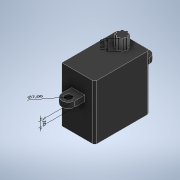
# Autodesk Inventor part: servo
Saved by Autodesk Inventor 2021 (Build 250183000, 183)
## iProperties
Created: 2021-02-24
Part Number: servo
Material: Rubber
Document SubType Name: Modeling
Designer: WASHINGTON
Density: 0.93 g/cm^3
Appearance: Rubber - Black
Author: WASHINGTON
Autodesk Inventor part; units mm, degrees
ref_plane "YZ Plane" through (0, 0, 0) normal (1, 0, 0) x (0, 1, 0)
ref_plane "XZ Plane" through (0, 0, 0) normal (0, 1, 0) x (-1, 0, 0)
ref_plane "XY Plane" through (0, 0, 0) normal (0, 0, 1) x (1, 0, 0)
sketch "Sketch1" plane through (0, 0, 0) normal (0, 1, 0) x (-1, 0, 0)
  line L0 (15, 25) -> (-15, 25)
  line L1 (-15, 25) -> (-15, -25)
  line L2 (-15, -25) -> (15, -25)
  line L3 (15, -25) -> (15, 25)
  circle A0 centre (0, -34) radius 3.5
  arc A1 (-6, -34) -> (6, -34) centre (0, -34) ccw
  line L4 (6, -34) -> (6, -25)
  line L5 (-6, -34) -> (-6, -25)
  line L6 (21.3749, 0) -> (-33.1106, 0) construction
  circle A2 centre (0, 34) radius 3.5
  arc A3 (6, 34) -> (-6, 34) centre (0, 34) ccw
  line L7 (6, 34) -> (6, 25)
  line L8 (-6, 34) -> (-6, 25)
  point P0 (0, 0)
  dimension "d0" = 25
  dimension "d1" = 25
  dimension "d2" = 15
  dimension "d3" = 15
  dimension "d4" = 7
  dimension "d5" = 12
  dimension "d6" = 9
  dimension "d7" = 34
  dimension "d8" = 12
  dimension "d9" = 34
  constraints: 18 end point, 6 symmetric about line, 4 centre point, 4 point on circle, 3 perpendicular, 2 coincident, 2 horizontal, 2 parallel, 2 point on line, 1 tangent, 2 other
  measures "d0" vertical distance of point (0, 0) L0.start
  measures "d1" distance from line of point (0, 0) L2
  measures "d2" horizontal distance of point (0, 0) L2.end
  measures "d3" horizontal distance of point (0, 0) L1.end
  measures "d4" diameter of A0
  measures "d5" diameter of A1
  measures "d6" distance from line of L2 A1.centre
  measures "d7" distance of point (0, 0) A0.centre
  measures "d8" distance between parallel lines of L5 L4
  measures "d9" distance of point (0, 0) A3.centre
extrude "Extrusion1" add sketch "Sketch1" along normal mid plane 5
sketch "Sketch2" plane through (0, 2.5, 0) normal (0, 1, 0) x (1, 0, 0)
  line L0 (-15, -25) -> (-15, 25) projected
  line L1 (6, 25) -> (15, 25) projected
  line L2 (-15, -25) -> (15, -25)
  line L3 (15, -25) -> (15, 25)
  line L4 (15, 25) -> (-15, 25)
  line L5 (-15, 25) -> (-15, -25)
  point P0 (0, 0)
  constraints: 8 end point, 2 parallel, 1 horizontal, 1 perpendicular
extrude "Extrusion2" add sketch "Sketch2" along normal blind 15 and the other way blind 35
sketch "Sketch3" plane through (0, 17.5, 0) normal (0, 1, 0) x (1, 0, 0)
  circle A0 centre (0, 15) radius 4
  line L0 (15, 25) -> (-15, 25) projected
  line L1 (-4, 15) -> (-5, 15) construction
  line L2 (-5, 15) -> (-5, 15.5)
  line L3 (-5, 15.5) -> (-3.8219, 16.1802)
  line L4 (-5, 15) -> (-5, 14.5)
  line L5 (-5, 14.5) -> (-3.8219, 13.8198)
  line L6 (-3.8891, 11.818) -> (-3.537, 13.132)
  line L7 (-3.5355, 11.4645) -> (-3.8891, 11.818)
  line L8 (-3.5355, 11.4645) -> (-3.182, 11.1109)
  line L9 (-3.182, 11.1109) -> (-1.868, 11.463)
  line L10 (-0.5, 10) -> (-1.1802, 11.1781)
  line L11 (0, 10) -> (-0.5, 10)
  line L12 (0, 10) -> (0.5, 10)
  line L13 (0.5, 10) -> (1.1802, 11.1781)
  line L14 (3.182, 11.1109) -> (1.868, 11.463)
  line L15 (3.5355, 11.4645) -> (3.182, 11.1109)
  line L16 (3.5355, 11.4645) -> (3.8891, 11.818)
  line L17 (3.8891, 11.818) -> (3.537, 13.132)
  line L18 (5, 14.5) -> (3.8219, 13.8198)
  line L19 (5, 15) -> (5, 14.5)
  line L20 (5, 15) -> (5, 15.5)
  line L21 (5, 15.5) -> (3.8219, 16.1802)
  line L22 (3.8891, 18.182) -> (3.537, 16.868)
  line L23 (3.5355, 18.5355) -> (3.8891, 18.182)
  line L24 (3.5355, 18.5355) -> (3.182, 18.8891)
  line L25 (3.182, 18.8891) -> (1.868, 18.537)
  line L26 (0.5, 20) -> (1.1802, 18.8219)
  line L27 (0, 20) -> (0.5, 20)
  line L28 (0, 20) -> (-0.5, 20)
  line L29 (-0.5, 20) -> (-1.1802, 18.8219)
  line L30 (-3.182, 18.8891) -> (-1.868, 18.537)
  line L31 (-3.5355, 18.5355) -> (-3.182, 18.8891)
  line L32 (-3.5355, 18.5355) -> (-3.8891, 18.182)
  line L33 (-3.8891, 18.182) -> (-3.537, 16.868)
  point P0 (0, 0)
  dimension "d16" = 8
  dimension "d17" = 10
  dimension "d18" = 15
  dimension "d19" = 120
  dimension "d20" = 0
  dimension "d21" = 1
  dimension "d22" = 0.5
  dimension "d25" = 360
  constraints: 66 end point, 2 point on circle, 2 symmetric about line, 1 centre point, 1 horizontal, 1 perpendicular, 73 other
  measures "d16" diameter of A0
  measures "d17" distance from line of L0 A0.centre
  measures "d18" distance of point (0, 0) A0.centre
  measures "d19" angle of L3 L2
  measures "d20" distance from line of A0.centre L1
  measures "d21" distance of L1.start L1.end
  measures "d22" distance of L1.end L2.end
extrude "Extrusion3" add sketch "Sketch3" along normal blind 10
fillet "Fillet1" radius 2 2 edges at (15, -7.5, 25) (15, -7.5, -25)
thread "Thread1" size "M7x1" class "6H" standard "ANSI Metric M Profile" full length
thread "Thread2" size "M7x1" class "6H" standard "ANSI Metric M Profile" full length
body "Solid1"
